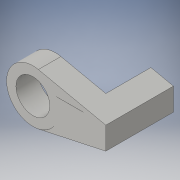
# Autodesk Inventor part: small pulley cable retainers
Saved by Autodesk Inventor 2016 (Build 200138000, 138)
## iProperties
Created: 2016-11-23
Part Number: small pulley cable retainers
Material: Generic
Document SubType Name: Modeling
Designer: paul_
Density: 1 g/cm^3
Appearance: Default
Author: paul_
## iProperties of the stored document small pulley cable retainers_3DPrint.ipt
Created: 2016-12-04
Part Number: small pulley cable retainers_3DPrint
Material: Generic
Document SubType Name: Modeling
Designer: paul_
Density: 1 g/cm^3
Appearance: Default
Author: paul_
Autodesk Inventor part; units mm, degrees
ref_plane "YZ Plane" through (0, 0, 0) normal (1, 0, 0) x (0, 1, 0)
ref_plane "XZ Plane" through (0, 0, 0) normal (0, 1, 0) x (-1, 0, 0)
ref_plane "XY Plane" through (0, 0, 0) normal (0, 0, 1) x (1, 0, 0)
sketch "Sketch1" plane through (0, 0, 0) normal (0, 0, 1) x (1, 0, 0)
  circle A0 centre (0, 0) radius 2.25
  arc A1 (3.165148, 1.493933) -> (3.159393, -1.506067) centre (0, 0) ccw
  line L0 (6.72439, -1.506067) -> (3.159393, -1.506067)
  line L1 (-0.27561, 3.050761) -> (6.72439, 3.050761) construction
  line L2 (1.598572, 1.503832) -> (1.673616, 1.503832)
  line L3 (3.165148, 1.493933) -> (6.72439, 1.493933)
  line L4 (6.72439, -1.506067) -> (6.72439, 1.493933)
  line L5 (6.72439, 1.493933) -> (6.72439, -1.506067)
  point P0 (7.357739, 0.5858)
  point P1 (6.72439, -0.006067)
  dimension "d0" = 4.5
  dimension "d1" = 7
  dimension "d3" = 7
  dimension "d13" = 3
  constraints: 12 end point, 3 horizontal, 2 coincident, 2 parallel, 2 perpendicular, 2 point on circle, 1 centre point, 1 midpoint, 3 other
  measures "d1" diameter of A1
  measures "d3" distance of L1.start L1.end
  measures "d13" distance of L3.end L0.start
extrude "Extrusion1" add sketch "Sketch1" along normal blind 3
sketch "Sketch2" plane through (0, 0, 0) normal (0, 0, -1) x (-1, 0, 0)
  line L0 (-6.708916, -1.496168) -> (-9.708916, -1.496168)
  line L1 (-9.708916, -1.496168) -> (-9.708916, 1.501612)
  line L2 (-9.708916, 1.501612) -> (-6.708916, 1.501612)
  line L3 (-6.708916, -1.496168) -> (-6.708916, 1.501612)
  line L4 (-3.159393, -1.506067) -> (-6.72439, -1.506067)
  point P0 (0, 0)
  point P1 (-9.708916, 0.002722)
  point P2 (-2.307375, -1.496168)
  point P3 (-6.72439, -1.506067)
  dimension "d7" = 3
  constraints: 8 end point, 4 point on line, 2 parallel, 1 horizontal, 1 midpoint, 1 perpendicular, 1 other
  measures "d7" distance of L0.start L0.end
extrude "Extrusion2" add sketch "Sketch2" along normal blind 6
sketch "Sketch6" plane through (0, 0, 0) normal (0, 0, 1) x (1, 0, 0)
  line L0 (6.708916, 1.501612) -> (9.708916, 1.501612)
  line L1 (9.708916, -1.496168) -> (6.72439, -1.496168)
  line L2 (6.710722, 1.501612) -> (9.708916, 1.501612)
  line L3 (9.708916, 1.501612) -> (9.708916, -1.496168)
  line L4 (9.708916, -1.496168) -> (6.710722, -1.496168)
  line L5 (6.710722, -1.496168) -> (6.710722, 1.501612)
  point P0 (0, 0)
  constraints: 8 end point, 2 parallel, 1 horizontal, 1 perpendicular
extrude "Extrusion5" add sketch "Sketch6" along normal blind 3
sketch "Sketch8" plane through (0, 0, 3) normal (0, 0, 1) x (1, 0, 0)
  line L0 (9.708916, -1.496168) -> (9.708916, 1.501612)
  line L1 (9.708916, 1.501612) -> (0.73239, 3.422514)
  line L2 (9.708916, -1.496168) -> (0.734374, -3.422089)
  arc A0 (3.165148, 1.493933) -> (0.73239, 3.422514) centre (0, 0) ccw
  line L3 (9.708916, 1.501612) -> (3.165148, 1.493933)
  line L4 (3.159385, -1.496168) -> (9.708916, -1.496168)
  arc A1 (0.734374, -3.422089) -> (3.159385, -1.496168) centre (0.024651, -0.038766) ccw
  point P0 (0, 0)
  point P1 (3.159393, -1.506067)
  point P2 (0.765599, -3.415388)
  constraints: 8 end point, 5 point on circle, 2 centre point, 1 horizontal, 1 point on line, 1 tangent
sketch "Sketch8 outline for Extrusion7" plane through (0, 0, 3) normal (0, 0, 1) x (1, 0, 0)
  line L0 (0.765599, -3.415388) -> (9.708916, -1.496168)
  arc A0 (3.159385, -1.496168) -> (0.765599, -3.415388) centre (0.024651, -0.038766) cw
  line L1 (9.708916, -1.496168) -> (3.159385, -1.496168)
  line L2 (3.165148, 1.493933) -> (9.708916, 1.501612)
  arc A1 (0.73239, 3.422514) -> (3.165148, 1.493933) centre (0, 0) cw
  line L3 (9.708916, 1.501612) -> (0.73239, 3.422514)
extrude "Extrusion7" add sketch "Sketch8 outline for Extrusion7" against normal blind 3
sketch "Sketch9" plane through (0, 0, 0) normal (0, 0, -1) x (-1, 0, 0)
  line L0 (-6.708916, -1.496168) -> (-6.708916, 1.501612)
  line L1 (-6.708916, 1.501612) -> (-6.708916, 2.143587)
  line L2 (-6.708916, 1.501612) -> (-9.708916, 1.501612)
  line L3 (-9.708916, 1.501612) -> (-6.708916, 2.143587)
  line L4 (-6.708916, 1.501612) -> (-9.708916, 1.501612)
  line L5 (-6.708916, -1.496168) -> (-6.708916, -2.139963)
  line L6 (-9.708916, -1.496168) -> (-0.765599, -3.415388)
  line L7 (-9.708916, -1.496168) -> (-6.708916, -1.496168)
  line L8 (-9.708916, -1.496168) -> (-6.708916, -1.496168)
  line L9 (-9.708916, -1.496168) -> (-6.708916, -2.139963)
  point P0 (0, 0)
  constraints: 12 end point, 3 collinear, 1 point on line, 1 vertical
extrude "Extrusion8" add sketch "Sketch9" along normal blind 6
body "Solid1"
